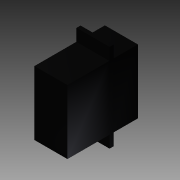
# Autodesk Inventor part: ServoMotor_SubSize
Saved by Autodesk Inventor 2014 SP1 (Build 180222100, 222)
## iProperties
Created: 2015-05-01
Part Number: ServoMotor_SubSize
Material: Generic
Document SubType Name: Modeling
Designer: david
Density: 1 g/cm^3
Appearance: Default
Author: david
Autodesk Inventor part; units mm, degrees
ref_plane "YZ Plane" through (0, 0, 0) normal (1, 0, 0) x (0, 1, 0)
ref_plane "XZ Plane" through (0, 0, 0) normal (0, 1, 0) x (-1, 0, 0)
ref_plane "XY Plane" through (0, 0, 0) normal (0, 0, 1) x (1, 0, 0)
sketch "Sketch1" plane through (0, 0, 0) normal (0, 1, 0) x (-1, 0, 0)
  line L0 (6.05, -11.7) -> (-6.05, -11.7)
  line L1 (-6.05, -11.7) -> (-6.05, 11.7)
  line L2 (-6.05, 11.7) -> (6.05, 11.7)
  line L3 (6.05, 11.7) -> (6.05, -11.7)
  line L4 (6.05, -11.7) -> (-6.05, 11.7) construction
  line L5 (-6.05, -11.7) -> (6.05, 11.7) construction
  point P0 (0, 0)
  dimension "d0" = 12.1
  dimension "d1" = 23.4
  constraints: 12 end point, 2 midpoint, 2 parallel, 1 horizontal, 1 perpendicular
  measures "d0" distance of L1.end L2.end
  measures "d1" distance of L0.end L1.end
extrude "Extrusion1" add sketch "Sketch1" along normal blind 25.8
sketch "Sketch2" plane through (-6.05, 0, 11.7) normal (0, 0, 1) x (1, 0, 0)
  line L0 (12.1, 0) -> (0, 0) projected
  line L1 (12.1, 0) -> (12.1, 25.8) projected
  line L2 (0, 0) -> (0, 25.8) projected
  line L3 (0, 16.9) -> (12.1, 16.9)
  line L4 (12.1, 16.9) -> (12.1, 15.4)
  line L5 (12.1, 15.4) -> (0, 15.4)
  line L6 (0, 15.4) -> (0, 16.9)
  point P0 (6.05, 0)
  dimension "d4" = 1.5
  dimension "d5" = 15.4
  constraints: 8 end point, 2 parallel, 2 point on line, 1 horizontal, 1 perpendicular
  measures "d4" distance between parallel lines of L5 L3
  measures "d5" distance between parallel lines of L0 L5
extrude "Extrusion2" add sketch "Sketch2" along normal blind 4.4 contours L5 L2 L3 L1
sketch "Sketch3" plane through (6.05, 0, -11.7) normal (0, 0, -1) x (-1, 0, 0)
  line L0 (12.1, 0) -> (0, 0) projected
  line L1 (12.1, 0) -> (12.1, 25.8) projected
  line L2 (0, 0) -> (0, 25.8) projected
  line L3 (0, 16.9) -> (12.1, 16.9)
  line L4 (12.1, 16.9) -> (12.1, 15.4)
  line L5 (12.1, 15.4) -> (0, 15.4)
  line L6 (0, 15.4) -> (0, 16.9)
  point P0 (6.05, 0)
  dimension "d8" = 1.5
  dimension "d9" = 15.4
  constraints: 8 end point, 2 parallel, 2 point on line, 1 horizontal, 1 perpendicular
  measures "d8" distance between parallel lines of L5 L3
  measures "d9" distance between parallel lines of L0 L5
extrude "Extrusion3" add sketch "Sketch3" along normal blind 4.4 contours L5 L2 L3 L1
sketch "Sketch4" plane through (0, 25.8, 0) normal (0, 1, 0) x (1, 0, 0)
  line L0 (-6.05, -11.7) -> (6.05, -11.7) projected
  line L1 (6.05, -11.7) -> (6.05, 11.7) projected
  circle A0 centre (0, -6.2) radius 2.35
  line L2 (0, 0) -> (0, -19.8821) construction
  dimension "d12" = 4.7
  dimension "d13" = 5.5
  constraints: 2 end point, 1 centre point, 1 parallel, 1 point on line
  measures "d12" diameter of A0
  measures "d13" distance from line of L0 A0.centre
extrude "Extrusion4" add sketch "Sketch4" along normal blind 2.8 separate body
body "Solid1"
body "Solid2"
